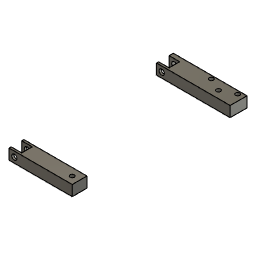
Стойки под управляющую рейку v11 (Autodesk Fusion 360 design; units mm, degrees)
Autodesk Fusion 360 part; units mm, degrees
sketch "Sketch1" plane through (0, 0, 0) normal (1, 0, 0) x (0, 0, -1)
  line L0 (0, 0) -> (-154, 0)
  line L1 (-154, 0) -> (-154, 10)
  line L2 (-154, 10) -> (0, 10)
  line L3 (0, 10) -> (0, 0)
  line L4 (-154, 10) -> (-140, 10)
  line L5 (-140, 10) -> (-140, 0)
  line L6 (-140, 0) -> (-154, 0)
  line L7 (-154, 0) -> (-154, 10)
  line L8 (0, 10) -> (-14, 10)
  line L9 (-14, 10) -> (-14, 0)
  line L10 (-14, 0) -> (0, 0)
  line L11 (0, 0) -> (0, 10)
  line L12 (-142, 10) -> (-152, 10)
  line L13 (-152, 10) -> (-152, 0)
  line L14 (-152, 0) -> (-142, 0)
  line L15 (-142, 0) -> (-142, 10)
  line L16 (-142, 10) -> (-152, 0) construction
  line L17 (-152, 10) -> (-142, 0) construction
  line L18 (-2, 10) -> (-12, 10)
  line L19 (-12, 10) -> (-12, 0)
  line L20 (-12, 0) -> (-2, 0)
  line L21 (-2, 0) -> (-2, 10)
  line L22 (-2, 10) -> (-12, 0) construction
  line L23 (-12, 10) -> (-2, 0) construction
  point P0 (-147, 5)
  point P1 (-7, 5)
  dimension "d2" = 10
  dimension "d3" = 14
  dimension "d4" = 10
  dimension "d5" = 14
  dimension "d6" = 10
  dimension "d7" = 10
  dimension "d8" = 10
  dimension "d9" = 10
  dimension "d10" = 10
  dimension "d11" = 2
  dimension "d12" = 2
  dimension "d38" = 10
  dimension "d39" = 10
  dimension "d40" = 126
  constraint horizontal L0
  constraint vertical L1
  constraint horizontal L2
  constraint vertical L3
  constraint coincident L0.start L3.end
  constraint horizontal L4
  constraint vertical L5
  constraint horizontal L6
  constraint vertical L7
  constraint horizontal L8
  constraint vertical L9
  constraint horizontal L10
  constraint vertical L11
  constraint horizontal L12
  constraint perpendicular L12 L13
  constraint parallel L12 L14
  constraint parallel L13 L15
  constraint coincident L16 P0
  constraint coincident L17 P0
  constraint horizontal L18
  constraint perpendicular L18 L19
  constraint parallel L18 L20
  constraint parallel L19 L21
  constraint coincident L22 P1
  constraint coincident L23 P1
  measures "d2" distance of L0.start L2.end
  measures "d3" distance of L1.end L4.end
  measures "d4" distance of L1.end L0.end
  measures "d5" distance of L2.end L8.end
  measures "d6" distance of L2 L10
  measures "d7" distance of L13.end L14.end
  measures "d8" distance of L12.end L13.end
  measures "d9" distance of L19.end L20.end
  measures "d10" distance of L18.end L19.end
  measures "d11" distance of L9 L19
  measures "d12" distance of L5 L15
  measures "d38" distance of L0 L18
  measures "d39" distance of L0 L12
  measures "d40" distance of L5 L9
extrude "Extrude1" add sketch "Sketch1" along normal blind 60 makes body 1
extrude "Extrude2" cut sketch "Sketch1" along normal blind 90 contours L0 L2 L5 L9 bodies 1 makes body 2 at (20, 0, 144.6667)
extrude "Extrude3" cut sketch "Sketch1" along normal blind 10 contours L0 L2 L8 L10 L18 L19 L20 L21 | L0 L2 L4 L6 L12 L13 L14 L15 bodies 1 2
sketch "Sketch4" plane through (0, 0, 154) normal (0, 0, 1) x (1, 0, 0)
  line L0 (0, 10) -> (0, 0)
  line L1 (0, 0) -> (60, 0)
  line L2 (60, 0) -> (60, 10)
  line L3 (60, 10) -> (0, 10)
  circle A0 centre (5, 5) radius 2.5
  dimension "d42" = 5
  measures "d42" diameter of A0
extrude "Extrude9" cut sketch "Sketch4" against normal blind 180 contours A0 bodies 1 2
sketch "Sketch5" plane through (0, 10, 0) normal (0, 1, 0) x (-1, 0, 0)
  line L0 (0, 2) -> (-10, 2)
  line L1 (-10, 2) -> (-10, 12)
  line L2 (-10, 12) -> (0, 12)
  line L3 (0, 12) -> (0, 14)
  line L4 (0, 14) -> (-60, 14)
  line L5 (-60, 14) -> (-60, 0)
  line L6 (-60, 0) -> (0, 0)
  line L7 (0, 0) -> (0, 2)
  circle A0 centre (-51.9439, 7) radius 2
  line L8 (-51.9439, 7) -> (-53, 147)
  circle A1 centre (-53, 147) radius 2
  dimension "d45" = 4
  dimension "d46" = 4
  constraint coincident A0.centre L8.start
  constraint coincident L8.end A1.centre
  measures "d45" diameter of A0
  measures "d46" diameter of A1
extrude "Extrude10" cut sketch "Sketch5" against normal blind 32 contours A0 | A1 bodies 1 2
extrude "Extrude11" add 1 faces at (42.5, 5, 154) along direction (0, 0, 1) blind 2 on bodies 2 bodies 2
extrude "Extrude12" cut 1 faces at (42.5, 5, 156) along direction (0, 0, -1) blind 2 on bodies 2 bodies 2
extrude "Extrude13" add 1 faces at (42.5, 5, 0) along direction (0, 0, -1) blind 2 on bodies 1 bodies 1
extrude "Extrude14" add 1 faces at (60, 3.3333, 3.3333) along direction (1, 0, 0) blind 10 on bodies 1 bodies 1
sketch "Sketch6" plane through (0, 10, 0) normal (0, 1, 0) x (-1, 0, 0)
  circle A0 centre (-51.9439, 7) radius 2
  line L0 (0, 2) -> (-10, 2)
  line L1 (-10, 2) -> (-10, 12)
  line L2 (-10, 12) -> (0, 12)
  line L3 (0, 12) -> (0, 14)
  line L4 (0, 14) -> (-70, 14)
  line L5 (-70, 14) -> (-70, -2)
  line L6 (-70, -2) -> (0, -2)
  line L7 (0, -2) -> (0, 2)
  line L8 (-70, -2) -> (-60, -2)
  line L9 (-60, -2) -> (-39.246, -2)
  line L10 (-39.246, -2) -> (-39.246, 1.042)
  circle A1 centre (-39.246, 1.042) radius 2
  line L11 (-39.246, 1.042) -> (-64.246, 1.042)
  circle A2 centre (-64.246, 1.042) radius 2
  dimension "d57" = 10
  dimension "d59" = 3.042
  dimension "d60" = 4
  dimension "d61" = 25
  dimension "d62" = 4
  dimension "d65" = 5.754
  constraint coincident L5.end L6.start
  constraint perpendicular L5 L8
  constraint perpendicular L5 L9
  constraint perpendicular L9 L10
  constraint coincident L10.end A1.centre
  constraint perpendicular L10 L11
  constraint coincident L11.end A2.centre
  measures "d57" distance of L5.end L8.end
  measures "d59" distance of L9.end L10.end
  measures "d60" diameter of A1
  measures "d61" distance of L10.end L11.end
  measures "d62" diameter of A2
  measures "d65" distance of L5 L11.end
extrude "Extrude15" cut sketch "Sketch6" against normal blind 32 contours L10 A1 L11 | L10 A1 L11 | A2 bodies 1
